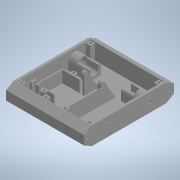
# Autodesk Inventor part: HexBody
Saved by Autodesk Inventor 2020 (Build 240168000, 168)
## iProperties
Created: 2023-12-19
Part Number: HexBody
Material: H TPU
Document SubType Name: Modeling
Designer: smz3rm
Density: 0.941117 g/cm^3
Appearance: Generic(1)
Mass: 177.509 g
Surface Area: 825.852 cm^2
Volume: 188.615 cm^3
BaseThickness: 3.000 mm
TopThickness: 1.778 mm
SideThickness: 4.000 mm
BodyWidth: 130.000 mm
BodyLength: 150.000 mm
BodyHeight: 30.000 mm
DriveMotorHeight: 15.000 mm
WheelWidth: 7.000 mm
WheelGrooveWidth: 4.000 mm
WheelGrooveDia: 16.000 mm
WheelDia: 40.000 mm
WheelPulleyDia: 2.000 mm
M3ScrewInsertBrim: 8.000 mm
M3ScrewDia: 3.100 mm
M3ScrewHeadDia: 6.100 mm
M3ScrewInsertDia: 4.000 mm
M3ScrewInsertDepth: 7.000 mm
DriveMotorOffset: 40.000 mm
DriveMotorHoleDia: 4.200 mm
M3ScrewHeadDepth: 2.200 mm
M3ScrewHeadTaper: -32.50 deg
WheeGuardlSlotWidth: 14.000 mm
WheelGuardScrewOffset: 7.000 mm
FlipperWidth: 20.000 mm
WheelSpokes: 5.000 ul
FlipperRodDia: 2.100 mm
FlipperArmThickness: 4.619 mm
FlipperArmLength: 87.010 mm
FlipperMountOffset: 70.000 mm
FlipperMountThickness: 6.000 mm
FlipperSpikeDrop: 37.509 mm
FlipperSpikeAngle: 30.00 deg
FlipperSpikeWidth: 10.000 mm
WheelGuardSpikeThickness: 8.000 mm
WheelGuardSpikeDrop: 35.200 mm
FlipperArmServoMountOffset: 30.000 mm
FlipperArmConnectorLength: 36.000 mm
VM3ScrewInsertDia: 3.750 mm
M2ScrewDia: 2.100 mm
Author: smz3rm
Autodesk Inventor part; units mm, degrees
ref_plane "XZ Plane" through (0, 0, 0) normal (0, 1, 0) x (-1, 0, 0)
ref_plane "XY Plane" through (0, 0, 0) normal (0, 0, 1) x (1, 0, 0)
sketch "Sketch1" plane through (0, 0, 0) normal (1, 0, 0) x (0, 1, 0)
  line L0 (-15, 75) -> (15, 75)
  line L1 (15, 75) -> (15, -75)
  line L2 (15, -75) -> (-15, -75)
  line L3 (-15, -75) -> (-15, 75)
  line L4 (-15, 75) -> (15, -75) construction
  line L5 (15, 75) -> (-15, -75) construction
  line L6 (-21, 0) -> (21, 0) projected
  line L7 (0, -105) -> (0, 105) projected
  line L8 (7.5, -75) -> (-7.5, -75)
  line L9 (-7.5, -75) -> (-15, -62.0096)
  line L10 (-15, -62.0096) -> (-7.5, -49.0192)
  line L11 (-7.5, -49.0192) -> (7.5, -49.0192)
  line L12 (7.5, -49.0192) -> (15, -62.0096)
  line L13 (15, -62.0096) -> (7.5, -75)
  line L14 (-7.5, 75) -> (-15, 62.0096)
  line L15 (15, 62.0096) -> (7.5, 75)
  point P0 (0, 0)
  point P1 (0, -62.0096)
  point P2 (7.5, 75)
  point P3 (-15, 62.0096)
  dimension "d0" = 30
  dimension "d1" = 150
  dimension "d25" = 12.9904
  constraints: 28 end point, 4 point on line, 4 symmetric about line, 2 midpoint, 2 parallel, 1 horizontal, 1 perpendicular, 13 other
  measures "d0" distance of L1.end L2.end
  measures "d1" distance of L0.end L1.end
  measures "d25" distance from line of point (0, -62.01) L2
extrude "Extrusion1" add sketch "Sketch1" along normal mid plane 130 contours L0 L7 L6 L3 L14 | L0 L15 L1 L6 L7 | L6 L7 L11 L10 L3 | L6 L1 L12 L11 L7 | L10 L11 L7 L2 L9 | L11 L12 L13 L2 L7
sketch "Sketch2" plane through (-65, 15, 62.4426) normal (0, 1, 0) x (1, 0, 0)
  line L0 (130, 124.4523) -> (130, 0.433) projected
  line L1 (0, 0.433) -> (0, 124.4523) projected
  line L2 (126, 124.4523) -> (4, 124.4523)
  line L3 (4, 124.4523) -> (4, 0.433)
  line L4 (4, 0.433) -> (126, 0.433)
  line L5 (126, 0.433) -> (126, 124.4523)
  line L6 (126, 124.4523) -> (4, 0.433) construction
  line L7 (4, 124.4523) -> (126, 0.433) construction
  line L8 (0, 0.433) -> (130, 0.433) projected
  line L9 (0, 124.4523) -> (130, 124.4523) projected
  line L10 (4, 124.0523) -> (126, 124.0523)
  line L11 (4, 0.833) -> (126, 0.833)
  point P0 (65, 62.4426)
  dimension "d4" = 4
  dimension "d89" = 0.4
  dimension "d90" = 0.4
  constraints: 16 end point, 5 point on line, 3 perpendicular, 2 midpoint, 2 parallel, 1 horizontal
  measures "d4" distance between parallel lines of L1 L3
  measures "d89" distance between parallel lines of L2 L10
  measures "d90" distance between parallel lines of L4 L11
extrude "Extrusion2" cut sketch "Sketch2" against normal blind 27 contours L5 L11 L3 L10
sketch "Sketch3" plane through (-65, -12, 62.4426) normal (0, 1, 0) x (1, 0, 0)
  line L0 (4, 0.833) -> (4, 124.0523) projected
  line L1 (126, 124.0523) -> (126, 0.833) projected
  line L2 (4, 0.833) -> (4, 124.0523) projected
  line L3 (126, 124.0523) -> (126, 0.833) projected
  line L4 (130, 124.4523) -> (130, 0.433) projected
  line L5 (0, 0.433) -> (0, 124.4523) projected
  line L6 (4, 124.0523) -> (12, 124.0523)
  line L7 (12, 124.0523) -> (12, 116.0523)
  line L8 (12, 116.0523) -> (4, 116.0523)
  line L9 (4, 116.0523) -> (4, 124.0523)
  line L10 (-26, 62.4426) -> (156, 62.4426) projected
  line L11 (65, 167.4426) -> (65, -42.5574) projected
  line L12 (118, 124.0523) -> (118, 116.0523)
  line L13 (118, 116.0523) -> (126, 116.0523)
  line L14 (12, 0.833) -> (12, 8.833)
  line L15 (12, 8.833) -> (4, 8.833)
  line L16 (118, 0.833) -> (118, 8.833)
  line L17 (118, 8.833) -> (126, 8.833)
  line L18 (0, 124.4523) -> (130, 124.4523) projected
  line L19 (0, 0.433) -> (130, 0.433) projected
  line L20 (126, 0.833) -> (4, 0.833) projected
  line L21 (4, 124.0523) -> (126, 124.0523) projected
  line L22 (126, 0.833) -> (4, 0.833) projected
  line L23 (4, 124.0523) -> (126, 124.0523) projected
  line L24 (4, 0.833) -> (4, 124.0523) projected
  line L25 (4, 124.0523) -> (126, 124.0523) projected
  point P0 (65, 62.4426)
  point P1 (4, 8.833)
  point P2 (126, 8.833)
  point P3 (12, 0.833)
  point P4 (12, 124.0523)
  point P5 (118, 124.0523)
  point P6 (118, 0.833)
  point P7 (118, 124.0523)
  point P8 (12, 124.0523)
  point P9 (12, 0.833)
  point P10 (118, 0.833)
  dimension "d8" = 8
  constraints: 20 end point, 9 symmetric about line, 2 horizontal, 2 parallel, 2 perpendicular, 1 collinear, 1 other
  measures "d8" distance of L7.end L8.end
extrude "Extrusion3" add sketch "Sketch3" along normal blind 25.222 contours L0 L15 L14 L20 | L0 L6 L7 L8 | L16 L17 L1 L20 | L13 L12 L21 L1
sketch "Sketch4" plane through (-61, 15, 62.0096) normal (1, 0, 0) x (0, 0, -1)
  circle A0 centre (97.0096, -15) radius 8.25
  line L0 (124.0192, -30) -> (0, -30) projected
  line L1 (137.0096, -7.5) -> (137.0096, -22.5) projected
  circle A1 centre (97.0096, -15) radius 10.25
  line L2 (86.7596, -15) -> (86.7596, -27)
  line L3 (8.4, -27) -> (115.6192, -27) projected
  line L4 (107.2596, -15) -> (107.2596, -27)
  point P0 (62.0096, -15)
  point P1 (0.4, -27)
  dimension "d12" = 16.5
  dimension "d13" = 15
  dimension "d14" = 40
  dimension "d15" = 2
  constraints: 4 end point, 2 centre point, 2 point on circle, 2 point on line, 2 tangent, 2 vertical, 1 coincident
  measures "d12" diameter of A0
  measures "d13" distance from line of L0 A0.centre
  measures "d14" distance from line of L1 A0.centre
  measures "d15" radial gap between concentric circles of A0 A1
extrude "Extrusion4" add sketch "Sketch4" along normal blind 14
sketch "Sketch5" plane through (-47, 15, 62.0096) normal (1, 0, 0) x (0, 0, -1)
  circle A0 centre (97.0096, -15) radius 8.25 projected
  circle A1 centre (97.0096, -15) radius 7.75
  arc A2 (107.2596, -15) -> (86.7596, -15) centre (97.0096, -15) ccw projected
  circle A3 centre (97.0096, -15) radius 8.25 projected
  line L0 (90.9096, -10.2196) -> (87.9426, -10.2196)
  arc A4 (107.2596, -15) -> (86.7596, -15) centre (97.0096, -15) ccw projected
  line L1 (90.9096, -10.2196) -> (90.9096, -27)
  line L2 (107.2596, -27) -> (86.7596, -27) projected
  line L3 (103.1096, -10.2196) -> (106.0766, -10.2196)
  line L4 (103.1096, -10.2196) -> (103.1096, -27)
  line L5 (86.7596, -15) -> (86.7596, -27) projected
  line L6 (107.2596, -27) -> (86.7596, -27) projected
  line L7 (107.2596, -27) -> (107.2596, -15) projected
  point P0 (62.0096, -15)
  point P1 (90.9096, -19.7804)
  point P2 (103.1096, -19.7804)
  dimension "d18" = 15.5
  dimension "d19" = 12.2
  constraints: 8 end point, 4 point on circle, 2 horizontal, 2 point on line, 1 centre point, 1 coincident, 1 parallel
  measures "d18" diameter of A1
  measures "d19" distance between parallel lines of L4 L1
extrude "Extrusion5" add sketch "Sketch5" along normal blind 20 contours A0 L4 A1 L3 | A0 L3 A2 L7 L2 L4 | L4 L2 L1 A0 | A0 L1 A1 L4 | L0 A1 L1 A0 | A0 L1 L2 L5 A2 L0 | A1 L4 | L1 A1
sketch "Sketch6" plane through (-61, 0, -35) normal (1, 0, 0) x (0, 0, -1)
  circle A0 centre (0, 0) radius 2.1
  point P0 (-35, 0)
  dimension "d22" = 4.2
  constraints: 1 centre point
  measures "d22" diameter of A0
extrude "Extrusion6" cut sketch "Sketch6" against normal through all
mirror "Mirror1" about plane through (0, 0, 0) normal (1, 0, 0) of "Extrusion4", "Extrusion5", "Extrusion6"
sketch "Sketch7" plane through (-65, 0, 0) normal (-1, 0, 0) x (0, 0, 1)
  line L0 (-105, 0) -> (105, 0) projected
  circle A0 centre (35, 0) radius 2
  line L1 (75, -7.5) -> (75, 7.5) projected
  point P0 (0, 0)
  dimension "d26" = 4
  dimension "d27" = 40
  constraints: 1 centre point, 1 point on line
  measures "d26" diameter of A0
  measures "d27" distance from line of L1 A0.centre
extrude "Extrusion7" cut sketch "Sketch7" against normal up to surface (4 mm away)
mirror "Mirror2" about plane through (0, 0, 0) normal (1, 0, 0) of "Extrusion7"
sketch "Sketch9" plane through (-65, 0, 0) normal (-1, 0, 0) x (0, 0, 1)
  line L0 (-75, -7.5) -> (-75, 7.5) projected
  line L1 (-75, 0) -> (-62.0096, 0)
  circle A0 centre (-68.5048, 0) radius 2
  line L2 (0, -21) -> (0, 21) projected
  circle A1 centre (68.5048, 0) radius 2
  line L3 (-75, -7.5) -> (-62.0096, -15) projected
  line L4 (-62.0096, -15) -> (-62.0096, 15)
  point P0 (0, 0)
  dimension "d30" = 4
  constraints: 4 end point, 4 midpoint, 2 centre point, 1 symmetric about line, 1 vertical, 1 other
  measures "d30" diameter of A0
extrude "Extrusion8" cut sketch "Sketch9" against normal blind 7 contours A0 L1 | L1 A0 | A1
mirror "Mirror3" about plane through (0, 0, 0) normal (1, 0, 0) of "Extrusion8"
ref_plane "Work Plane1" through (11, 0, 0) normal (1, 0, 0) x (0, 1, 0)
sketch "Sketch10" plane through (11, 0, 0) normal (1, 0, 0) x (0, 1, 0)
  line L0 (-12, 61.6096) -> (-12, -24.75) projected
  line L1 (-12, -1.4782) -> (20.3594, -1.4782)
  line L2 (20.3594, -1.4782) -> (20.3594, -6.7609)
  line L3 (20.3594, -6.7609) -> (-12, -25.4436)
  circle A0 centre (17.3094, -5) radius 1.05
  line L4 (-7.5, -75) -> (7.5, -75) projected
  line L5 (15, -62.0096) -> (15, 62.0096) projected
  line L6 (-12, -24.75) -> (-12, -45.25) projected
  line L7 (-12, -61.6096) -> (-12, 53.6096) projected
  line L8 (20.3594, -6.7609) -> (17.3094, -8.5218)
  line L9 (17.3094, -8.5218) -> (14.2594, -6.7609)
  line L10 (14.2594, -6.7609) -> (14.2594, -3.2391)
  line L11 (14.2594, -3.2391) -> (17.3094, -1.4782)
  line L12 (17.3094, -1.4782) -> (20.3594, -3.2391)
  line L13 (20.3594, -3.2391) -> (20.3594, -6.7609)
  point P0 (0, 0)
  point P1 (18.3594, -5)
  point P2 (15, -9.8552)
  point P3 (15, -1.4782)
  point P4 (-12, -53.6096)
  dimension "d34" = 2.1
  dimension "d38" = 70
  dimension "d40" = 1.05
  dimension "d41" = 2.3094
  dimension "d44" = 60
  dimension "d45" = 2
  constraints: 18 end point, 4 point on line, 1 coincident, 1 collinear, 1 horizontal, 1 horizontal alignment, 1 perpendicular, 15 other
  measures "d38" distance from line of L4 point (17.309, -5)
  measures "d40" distance of point (17.309, -5) point (18.359, -5)
  measures "d41" distance from line of L5 point (17.309, -5)
  measures "d44" angle of L0 L3
  measures "d45" distance from line of L13 point (18.359, -5)
extrude "Extrusion9" add sketch "Sketch10" along normal blind 6 contours L1 L5 L11 L10 L9 L3 L6 L0 | L1 L11 L5 | L12 L2 L3 L9 L5 L11 | L5 L9 L10 L11 | L5 L9 L3
mirror "Mirror4" about plane through (0, 0, 0) normal (1, 0, 0) of "Extrusion9"
sketch "Sketch12" plane through (-65, -12, 62.4426) normal (0, 1, 0) x (1, 0, 0)
  line L0 (126, 116.0523) -> (126, 107.6926) projected
  line L1 (126, 116.0523) -> (118, 116.0523) projected
  line L2 (118, 116.0523) -> (118, 124.0523) projected
  line L3 (12, 124.0523) -> (12, 116.0523) projected
  line L4 (12, 116.0523) -> (4, 116.0523) projected
  line L5 (4, 107.6926) -> (4, 116.0523) projected
  line L6 (4, 8.833) -> (12, 8.833) projected
  line L7 (12, 8.833) -> (12, 0.833) projected
  line L8 (118, 0.833) -> (118, 8.833) projected
  line L9 (118, 8.833) -> (126, 8.833) projected
  line L10 (53, 0.833) -> (45, 0.833)
  line L11 (45, 0.833) -> (45, 8.833)
  line L12 (45, 8.833) -> (53, 8.833)
  line L13 (53, 8.833) -> (53, 0.833)
  line L14 (65, 167.4426) -> (65, -42.5574) projected
  line L15 (85, 0.833) -> (85, 8.833)
  line L16 (85, 8.833) -> (77, 8.833)
  line L17 (77, 8.833) -> (77, 0.833)
  line L18 (12, 124.0523) -> (118, 124.0523) projected
  line L19 (118, 0.833) -> (12, 0.833) projected
  line L20 (126, 87.1926) -> (92, 87.1926) projected
  line L21 (92, 87.1926) -> (92, 107.6926) projected
  line L22 (92, 107.6926) -> (126, 107.6926) projected
  line L23 (4, 107.6926) -> (38, 107.6926) projected
  line L24 (38, 107.6926) -> (38, 87.1926) projected
  line L25 (38, 87.1926) -> (4, 87.1926) projected
  line L26 (4, 8.833) -> (4, 87.1926) projected
  line L27 (126, 87.1926) -> (126, 8.833) projected
  line L28 (82, 63.9208) -> (76, 63.9208) projected
  line L29 (54, 63.9208) -> (48, 63.9208) projected
  line L30 (76, 63.9208) -> (82, 63.9208) projected
  line L31 (54, 63.9208) -> (48, 63.9208) projected
  point P0 (65, 62.4426)
  point P1 (77, 0.833)
  point P2 (85, 0.833)
  dimension "d46" = 8
  dimension "d55" = 12
  constraints: 14 end point, 4 symmetric about line, 2 parallel, 2 perpendicular, 1 collinear, 1 horizontal
  measures "d46" distance of L11.end L12.end
  measures "d55" distance between parallel lines of L14 L13
extrude "Extrusion10" add sketch "Sketch12" along normal blind 25.222 contours L17 L16 L15 L19 | L10 L11 L12 L13
sketch "Sketch13" plane through (-65, 13.222, 62.4426) normal (0, 1, 0) x (1, 0, 0)
  line L0 (12, 116.0523) -> (12, 124.0523) projected
  line L1 (4, 124.0523) -> (12, 124.0523) projected
  line L2 (4, 116.0523) -> (4, 124.0523) projected
  line L3 (4, 116.0523) -> (12, 116.0523) projected
  line L4 (118, 124.0523) -> (126, 124.0523) projected
  line L5 (118, 124.0523) -> (118, 116.0523) projected
  line L6 (118, 116.0523) -> (126, 116.0523) projected
  line L7 (126, 124.0523) -> (126, 116.0523) projected
  line L8 (12, 0.833) -> (4, 0.833) projected
  line L9 (12, 0.833) -> (12, 8.833) projected
  line L10 (12, 8.833) -> (4, 8.833) projected
  line L11 (4, 0.833) -> (4, 8.833) projected
  line L12 (53, 0.833) -> (45, 0.833) projected
  line L13 (53, 0.833) -> (53, 8.833) projected
  line L14 (53, 8.833) -> (45, 8.833) projected
  line L15 (45, 8.833) -> (45, 0.833) projected
  line L16 (126, 8.833) -> (126, 0.833) projected
  line L17 (126, 8.833) -> (118, 8.833) projected
  line L18 (118, 8.833) -> (118, 0.833) projected
  line L19 (126, 0.833) -> (118, 0.833) projected
  line L20 (85, 0.833) -> (85, 8.833) projected
  line L21 (85, 8.833) -> (77, 8.833) projected
  line L22 (77, 8.833) -> (77, 0.833) projected
  line L23 (85, 0.833) -> (77, 0.833) projected
  circle A0 centre (8, 120.0523) radius 1.875
  line L24 (4, 116.0523) -> (4, 124.0523) projected
  line L25 (4, 120.0523) -> (12, 120.0523)
  line L26 (4, 124.0523) -> (12, 124.0523) projected
  line L27 (8, 124.0523) -> (8, 116.0523)
  line L28 (12, 116.0523) -> (4, 116.0523) projected
  line L29 (-26, 62.4426) -> (156, 62.4426) projected
  line L30 (65, 167.4426) -> (65, -42.5574) projected
  circle A1 centre (122, 120.0523) radius 1.875
  circle A2 centre (8, 4.833) radius 1.875
  circle A3 centre (122, 4.833) radius 1.875
  circle A4 centre (49, 4.833) radius 1.875
  line L31 (45, 0.833) -> (45, 8.833) projected
  line L32 (45, 4.833) -> (53, 4.833)
  line L33 (53, 8.833) -> (45, 8.833) projected
  line L34 (49, 8.833) -> (49, 0.833)
  circle A5 centre (81, 4.833) radius 1.875
  dimension "d91" = 3.75
  dimension "d92" = 3.75
  constraints: 10 midpoint, 8 end point, 6 centre point, 4 symmetric about line, 4 other
  measures "d91" diameter of A0
  measures "d92" diameter of A4
extrude "Extrusion11" cut sketch "Sketch13" against normal blind 7 contours L25 L27 A0 | A0 L27 L25 | A0 L25 L27 | L27 L25 A0 | L34 L32 A4 | A4 L32 L34 | L32 L34 A4 | A4 L34 L32 | A1 | A2 | A3 | A5
sketch "Sketch14" plane through (-65, -12, 62.4426) normal (0, 1, 0) x (1, 0, 0)
  line L0 (17.5, 63.9208) -> (58, 63.9208)
  line L1 (58, 63.9208) -> (58, 22.9208)
  line L2 (58, 22.9208) -> (17.5, 22.9208)
  line L3 (17.5, 22.9208) -> (17.5, 63.9208)
  line L4 (60, 65.9208) -> (15.5, 65.9208)
  line L5 (15.5, 65.9208) -> (15.5, 20.9208)
  line L6 (15.5, 20.9208) -> (60, 20.9208)
  line L7 (60, 20.9208) -> (60, 65.9208)
  line L8 (48, 63.9208) -> (48, 20.9208)
  line L9 (46, 65.9208) -> (46, 20.9208)
  line L10 (36.3688, 67.9208) -> (34.0594, 63.9208)
  line L11 (34.0594, 63.9208) -> (29.4406, 63.9208)
  line L12 (29.4406, 63.9208) -> (27.1312, 67.9208)
  line L13 (27.1312, 67.9208) -> (29.4406, 71.9208)
  line L14 (29.4406, 71.9208) -> (34.0594, 71.9208)
  line L15 (34.0594, 71.9208) -> (36.3688, 67.9208)
  line L16 (17.5, 63.9208) -> (46, 63.9208)
  line L17 (31.75, 63.9208) -> (31.75, 67.9208)
  line L18 (15.5, 43.4208) -> (60, 43.4208)
  line L19 (36.3688, 18.9208) -> (34.0594, 22.9208)
  line L20 (34.0594, 22.9208) -> (29.4406, 22.9208)
  line L21 (29.4406, 22.9208) -> (27.1312, 18.9208)
  line L22 (27.1312, 18.9208) -> (29.4406, 14.9208)
  line L23 (29.4406, 14.9208) -> (34.0594, 14.9208)
  line L24 (34.0594, 14.9208) -> (36.3688, 18.9208)
  line L25 (21.5, 22.9208) -> (26, 22.9208)
  line L26 (26, 22.9208) -> (26, 20.9208)
  line L27 (26, 20.9208) -> (21.5, 20.9208)
  line L28 (21.5, 20.9208) -> (21.5, 22.9208)
  point P0 (65, 62.4426)
  point P1 (31.75, 18.9208)
  point P2 (36.8688, 67.3434)
  point P3 (27.6312, 67.3434)
  point P4 (27.6312, 19.3434)
  point P5 (36.8688, 19.3434)
  point P6 (46, 22.9208)
  point P7 (28.2859, 65.9208)
  point P8 (35.2141, 65.9208)
  point P9 (35.2141, 20.9208)
  point P10 (28.2859, 20.9208)
  point P11 (29.4406, 22.9208)
  point P12 (29.4406, 63.9208)
  point P13 (29.4406, 22.9208)
  point P14 (34.0594, 22.9208)
  point P15 (34.0594, 22.9208)
  point P16 (26, 22.9208)
  dimension "d56" = 30.5
  dimension "d57" = 41
  dimension "d58" = 40.5
  dimension "d59" = 2
  dimension "d60" = 2
  dimension "d62" = 8
  dimension "d102" = 4.5
  dimension "d104" = 8.5
  constraints: 58 end point, 8 point on line, 7 symmetric about line, 6 parallel, 5 perpendicular, 3 midpoint, 2 horizontal, 1 collinear, 1 vertical, 16 other
  measures "d56" distance of L8.start L0.start
  measures "d57" distance of L2.end L0.start
  measures "d58" distance of L1.end L2.end
  measures "d59" distance between parallel lines of L0 L4
  measures "d60" distance between parallel lines of L8 L9
  measures "d62" distance between parallel lines of L11 L14
  measures "d102" distance of L26.end L27.end
  measures "d104" distance between parallel lines of L3 L26
extrude "Extrusion12" add sketch "Sketch14" along normal blind 19.5 contours L3 L18 L5 L4 L12 L0 | L12 L4 L17 L0 | L3 L2 L28 L6 L5 L18 | L17 L4 L10 L0 | L12 L13 L14 L15 L10 L4 | L10 L4 L9 L0 | L9 L6 L19 L2 | L2 L21 L6 L26 | L19 L6 L21 L2 | L19 L24 L23 L22 L21 L6
sketch "Sketch15" plane through (-65, 7.5, 62.4426) normal (0, 1, 0) x (1, 0, 0)
  line L0 (15.5, 20.9208) -> (21.5, 20.9208) projected
  line L1 (28.2859, 65.9208) -> (15.5, 65.9208) projected
  line L2 (46, 65.9208) -> (35.2141, 65.9208) projected
  line L3 (15.5, 65.9208) -> (15.5, 20.9208) projected
  circle A0 centre (31.75, 67.9208) radius 1.875
  circle A1 centre (31.75, 18.9208) radius 1.875
  line L4 (29.4406, 71.9208) -> (27.1312, 67.9208) projected
  line L5 (35.2141, 65.9208) -> (36.3688, 67.9208) projected
  line L6 (36.3688, 67.9208) -> (34.0594, 71.9208) projected
  line L7 (34.0594, 71.9208) -> (29.4406, 71.9208) projected
  line L8 (29.4406, 71.9208) -> (27.1312, 67.9208) projected
  line L9 (27.1312, 67.9208) -> (28.2859, 65.9208) projected
  line L10 (28.2859, 20.9208) -> (27.1312, 18.9208) projected
  line L11 (27.1312, 18.9208) -> (29.4406, 14.9208) projected
  line L12 (29.4406, 14.9208) -> (34.0594, 14.9208) projected
  line L13 (34.0594, 14.9208) -> (36.3688, 18.9208) projected
  line L14 (36.3688, 18.9208) -> (35.2141, 20.9208) projected
  line L15 (35.2141, 20.9208) -> (46, 20.9208) projected
  line L16 (36.3688, 67.9208) -> (27.1312, 67.9208)
  line L17 (27.1312, 18.9208) -> (28.2859, 20.9208) projected
  line L18 (36.3688, 18.9208) -> (34.0594, 14.9208) projected
  line L19 (27.1312, 18.9208) -> (36.3688, 18.9208)
  line L20 (46, 20.9208) -> (46, 22.9208) projected
  line L21 (46, 22.9208) -> (26, 22.9208) projected
  line L22 (26, 22.9208) -> (26, 20.9208) projected
  line L23 (26, 20.9208) -> (28.2859, 20.9208) projected
  line L24 (21.5, 20.9208) -> (21.5, 22.9208) projected
  line L25 (21.5, 22.9208) -> (17.5, 22.9208) projected
  line L26 (17.5, 22.9208) -> (17.5, 63.9208) projected
  line L27 (17.5, 63.9208) -> (46, 63.9208) projected
  line L28 (46, 63.9208) -> (46, 65.9208) projected
  point P0 (65, 62.4426)
  point P1 (27.6312, 67.3434)
  dimension "d66" = 3.75
  constraints: 4 end point, 2 centre point, 2 midpoint, 1 equal radius, 1 horizontal, 1 other
  measures "d66" diameter of A1
extrude "Extrusion13" cut sketch "Sketch15" against normal blind 7 contours L16 A0 | A0 L16 | L19 A1 | A1 L19
sketch "Sketch16" plane through (-17, -12, -1.4782) normal (-1, 0, 0) x (0, 0, 1)
  line L0 (0, 29.3094) -> (0, 0) projected
  line L1 (0, 0) -> (-23.9655, 0) projected
  line L2 (0, 20) -> (-7.5, 20)
  line L3 (-7.5, 20) -> (-7.5, 0)
  line L4 (-7.5, 0) -> (0, 0)
  line L5 (0, 0) -> (0, 20)
  point P0 (1.4782, 12)
  dimension "d69" = 20
  dimension "d70" = 7.5
  constraints: 8 end point, 2 parallel, 2 point on line, 1 horizontal, 1 perpendicular
  measures "d69" distance of L4.end L2.start
  measures "d70" distance of L2.start L2.end
extrude "Extrusion14" cut sketch "Sketch16" against normal blind 3
sketch "Sketch20" plane through (-61, 15, 61.6096) normal (1, 0, 0) x (0, 0, -1)
  circle A0 centre (26.6096, -15) radius 2 projected
  line L0 (22.6096, -27) -> (30.6096, -27)
  line L1 (30.6096, -27) -> (30.6096, -11)
  line L2 (30.6096, -11) -> (22.6096, -11)
  line L3 (22.6096, -11) -> (22.6096, -27)
  line L4 (8, -27) -> (86.3596, -27) projected
  line L5 (26.6096, -11) -> (26.6096, -15)
  point P0 (61.6096, -15)
  dimension "d96" = 8
  dimension "d97" = 4
  constraints: 10 end point, 2 parallel, 1 horizontal, 1 midpoint, 1 perpendicular, 1 point on line, 1 vertical
  measures "d96" distance of L1.end L2.end
  measures "d97" distance from line of L2 L5.end
extrude "Extrusion17" add sketch "Sketch20" along normal blind 3
sketch "Sketch21" plane through (-11, -12, -1.4782) normal (0, 0, 1) x (1, 0, 0)
  line L0 (-6, 20) -> (-3, 20) projected
  line L1 (-3, 20) -> (-6, 23)
  line L2 (-3, 20) -> (1.2426, 20) construction
  line L3 (-6, 29.3094) -> (-6, 20) projected
  point P0 (11, 12)
  dimension "d105" = 135
  constraints: 4 end point, 1 equal length, 1 horizontal, 1 point on line
  measures "d105" angle of L2 L1
extrude "Extrusion18" cut sketch "Sketch21" against normal up to surface (7.5 mm away)
mirror "Mirror6" about plane through (0, 0, 0) normal (1, 0, 0) of "Extrusion17"
sketch "Sketch22" plane through (-17, 20.3594, -6.7609) normal (-1, 0, 0) x (0, 0, 1)
  circle A0 centre (1.7609, -3.05) radius 1.05 projected
  point P0 (6.7609, -20.3594)
extrude "Extrusion19" add sketch "Sketch22" against normal blind 1
mirror "Mirror7" about plane through (0, 0, 0) normal (1, 0, 0) of "Extrusion19"
sketch "Sketch23" plane through (-65, -12, 62.4426) normal (0, 1, 0) x (1, 0, 0)
  line L0 (82, 63.9208) -> (81.2, 63.9208)
  line L1 (81.2, 63.9208) -> (81.2, 8.833)
  line L2 (81.2, 8.833) -> (82, 8.833)
  line L3 (82, 8.833) -> (82, 63.9208)
  line L4 (85, 8.833) -> (77, 8.833) projected
  dimension "d110" = 0.8
  constraints: 8 end point, 2 parallel, 1 coincident, 1 horizontal, 1 perpendicular, 1 point on line
  measures "d110" distance of L2.end L1.end
extrude "Extrusion20" add sketch "Sketch23" along normal up to surface (25.222 mm away)
equation "\"d0\" = BodyHeight"
equation "\"d1\" = BodyLength"
equation "\"d2\" = BodyWidth"
equation "\"d4\" = SideThickness"
equation "\"d5\" = BodyHeight - BaseThickness"
equation "\"d8\" = M3ScrewInsertBrim"
equation "\"d10\" = -BaseThickness + BodyHeight - TopThickness"
equation "\"d13\" = DriveMotorHeight"
equation "\"d14\" = DriveMotorOffset"
equation "\"d22\" = DriveMotorHoleDia"
equation "\"d26\" = M3ScrewInsertDia"
equation "\"d27\" = DriveMotorOffset"
equation "\"d30\" = M3ScrewInsertDia"
equation "\"d31\" = M3ScrewInsertDepth"
equation "\"d38\" = FlipperMountOffset"
equation "\"d40\" = 0.5 * d34"
equation "\"d41\" = 0.5 * FlipperArmThickness"
equation "\"d42\" = FlipperMountThickness"
equation "\"d46\" = M3ScrewInsertBrim"
equation "\"d48\" = -BaseThickness + BodyHeight - TopThickness"
equation "\"d53\" = M3ScrewInsertDepth"
equation "\"BaseThickness\" = 3"
equation "\"TopThickness\" = 1.778"
equation "\"SideThickness\" = 4"
equation "\"BodyWidth\" = 130"
equation "\"BodyLength\" = 150"
equation "\"BodyHeight\" = 30"
equation "\"DriveMotorHeight\" = 0.5 * BodyHeight"
equation "\"WheelWidth\" = 7"
equation "\"WheelGrooveWidth\" = 4"
equation "\"WheelGrooveDia\" = 0.4 * WheelDia"
equation "\"WheelPulleyDia\" = 2"
equation "\"M3ScrewInsertBrim\" = 8"
equation "\"M3ScrewDia\" = 3.1"
equation "\"M3ScrewHeadDia\" = 6.1"
equation "\"M3ScrewInsertDia\" = 4"
equation "\"M3ScrewInsertDepth\" = 7"
equation "\"DriveMotorOffset\" = 40"
equation "\"DriveMotorHoleDia\" = 4.2"
equation "\"M3ScrewHeadDepth\" = 2.2"
equation "\"M3ScrewHeadTaper\" = -32.5deg"
equation "\"WheelGuardScrewOffset\" = 7"
equation "\"FlipperArmLength\" = 2.5 * M3ScrewInsertBrim - FlipperMountOffset + BodyLength - 0.433013 * BodyHeight"
equation "\"FlipperWidth\" = 20"
equation "\"WheelSpokes\" = 5"
equation "\"FlipperRodDia\" = 2.1"
equation "\"FlipperMountOffset\" = 70"
equation "\"FlipperMountThickness\" = 6"
equation "\"FlipperSpikeWidth\" = 10"
equation "\"FlipperSpikeAngle\" = 30deg"
equation "\"WheelGuardSpikeThickness\" = 8"
equation "\"FlipperArmServoMountOffset\" = 30"
equation "\"FlipperArmConnectorLength\" = 36"
equation "\"VM3ScrewInsertDia\" = 3.75"
equation "\"M2ScrewDia\" = 2.1"
equation "\"WheelDia\" = 40"
equation "\"FlipperArmThickness\" = 4.618802"
body "Solid1"
